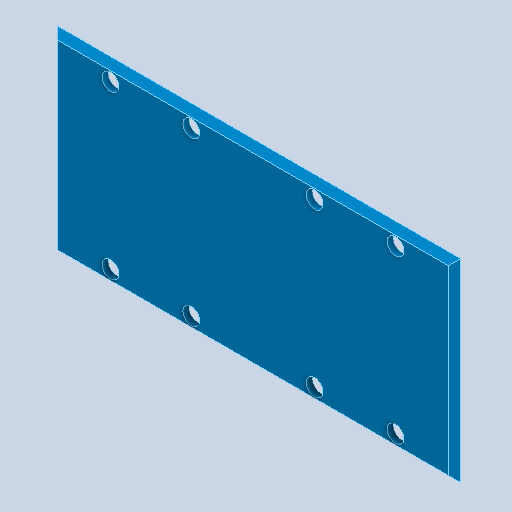
# Autodesk Inventor part: Panel Height 1x2
Saved by Autodesk Inventor 2023.1 (Build 271208000, 208)
## iProperties
Created: 2022-08-10
Part Number: Panel Height 1x2
Material: Generic
Document SubType Name: Modeling
Designer: xSibe
Density: 1 g/cm^3
Appearance: Plastic Teal
Author: xSibe
Autodesk Inventor part; units mm, degrees
ref_plane "YZ Plane" through (0, 0, 0) normal (1, 0, 0) x (0, 1, 0)
ref_plane "XZ Plane" through (0, 0, 0) normal (0, 1, 0) x (-1, 0, 0)
sketch "Sketch1" plane through (0, 0, 0) normal (0, 0, 1) x (1, 0, 0)
  line L0 (49.8, -22.9) -> (49.8, 22.9) projected
  line L1 (42.1, 24.9) -> (0.75, 24.9) projected
  line L2 (0.75, -24.9) -> (42.1, -24.9) projected
  line L3 (0, 22.9) -> (0, -22.9) projected
  line L4 (0.75, -22.9) -> (0.75, 22.9) projected
  line L5 (42.1, -22.9) -> (0.75, -22.9) projected
  line L6 (42.1, -22.9) -> (42.1, -17.05) projected
  line L7 (7.7, -17.05) -> (42.1, -17.05) projected
  line L8 (7.7, 17.05) -> (7.7, -17.05) projected
  line L9 (7.7, 17.05) -> (42.1, 17.05) projected
  line L10 (42.1, 17.05) -> (42.1, 22.9) projected
  line L11 (0.75, 22.9) -> (42.1, 22.9) projected
  circle A0 centre (34.8, -19.9) radius 2.0625 projected
  circle A1 centre (34.8, 19.9) radius 2.0625 projected
  circle A2 centre (15, -19.9) radius 2.0625 projected
  circle A3 centre (15, 19.9) radius 2.0625 projected
  line L12 (24.9, 17.05) -> (24.9, -17.05)
  line L13 (-0.1, 23.75) -> (49.9, 23.75)
  line L14 (49.9, 23.75) -> (49.9, -23.75)
  line L15 (49.9, -23.75) -> (-0.1, -23.75)
  line L16 (-0.1, -23.75) -> (-0.1, 23.75)
  line L17 (-0.1, 23.75) -> (49.9, -23.75) construction
  line L18 (49.9, 23.75) -> (-0.1, -23.75) construction
  point P0 (0, 0)
  point P1 (24.9, 0)
  dimension "d0" = 50
  dimension "d1" = 47.5
  constraints: 14 end point, 5 midpoint, 2 parallel, 1 horizontal, 1 perpendicular
  measures "d0" distance of L14.end L15.end
  measures "d1" distance of L13.end L14.end
ref_plane "Work Plane1" through (0.75, -22.9, 24.9) normal (0, 0, 1) x (1, 0, 0)
extrude "Extrusion1" add sketch "Sketch1" along normal blind 1.5 from surface at 24.9 contours L4 L11 L10 L9 L8 L7 L6 L5 | L7 L8 L9 L12 | L13 L14 L15 L16
pattern_linear "Rectangular Pattern1" count 2 spacing 50 along (1, 0, 0) of "Extrusion1"
sketch "Sketch2" plane through (-0.1, -23.75, 26.4) normal (0, 0, 1) x (1, 0, 0)
  circle A0 centre (65.1, 43.65) radius 2.0625 projected
  circle A1 centre (84.9, 43.65) radius 2.0625 projected
  circle A2 centre (84.9, 3.85) radius 2.0625 projected
  circle A3 centre (65.1, 3.85) radius 2.0625 projected
  line L0 (0, 0) -> (0, 47.5) projected
  line L1 (100, 0) -> (0, 0) projected
  line L2 (100, 47.5) -> (100, 0) projected
  line L3 (0, 47.5) -> (100, 47.5) projected
  circle A4 centre (15.1, 3.85) radius 2.0625 projected
  circle A5 centre (34.9, 3.85) radius 2.0625 projected
  circle A6 centre (34.9, 43.65) radius 2.0625 projected
  circle A7 centre (15.1, 43.65) radius 2.0625 projected
  line L4 (50, 47.5) -> (50, 0)
  line L5 (0.625, 0) -> (99.375, 0)
  line L6 (99.375, 0) -> (99.375, 47.5)
  line L7 (99.375, 47.5) -> (0.625, 47.5)
  line L8 (0.625, 47.5) -> (0.625, 0)
  line L9 (0.625, 0) -> (99.375, 47.5) construction
  line L10 (99.375, 0) -> (0.625, 47.5) construction
  point P0 (0.1, 23.75)
  point P1 (50, 23.75)
  point P2 (0.625, 47.5)
  dimension "d10" = 98.75
  constraints: 14 end point, 5 midpoint, 2 parallel, 1 horizontal, 1 perpendicular, 1 point on line
  measures "d10" distance of L7.end L6.end
extrude "Extrusion2" cut sketch "Sketch2" against normal up to surface (1.5 mm away) contours L0 L3 L8 L1 | L6 L3 L2 L1
chamfer "Chamfer1" distance 1.5 angle 45 4 edges at (49.9, 23.75, 26.4) (49.9, -23.75, 26.4) (99.275, 0, 26.4) (0.525, 0, 26.4)
body "Solid1"
